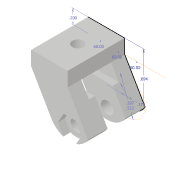
# Autodesk Inventor part: omni wheel wheel holder tilted
Saved by Autodesk Inventor 2018 (Build 220112000, 112)
## iProperties
Created: 2019-01-03
Part Number: omni wheel wheel holder tilted
Material: Generic
Document SubType Name: Modeling
Designer: ball
Density: 1 g/cm^3
Appearance: Default
Author: ball
Autodesk Inventor part; units mm, degrees
ref_plane "YZ Plane" through (0, 0, 0) normal (1, 0, 0) x (0, 1, 0)
ref_plane "XZ Plane" through (0, 0, 0) normal (0, 1, 0) x (-1, 0, 0)
ref_plane "XY Plane" through (0, 0, 0) normal (0, 0, 1) x (1, 0, 0)
sketch "Sketch1" plane through (0, 0, 0) normal (0, 0, 1) x (1, 0, 0)
  line L0 (6.5024, 17.6276) -> (-6.5024, 17.6276)
  line L1 (-6.5024, 12.5476) -> (6.5024, 12.5476) construction
  line L2 (6.5024, 12.5476) -> (13.7468, 0)
  line L3 (6.5024, 12.5476) -> (20.9911, 12.5476) construction
  line L4 (-6.5024, 12.5476) -> (0.742, 0)
  line L5 (-6.5024, 12.5476) -> (7.9863, 12.5476) construction
  line L6 (0, 12.5476) -> (7.2444, 0) construction
  line L7 (0, 12.5476) -> (14.4887, 12.5476) construction
  circle A0 centre (7.2444, 0) radius 2.1844
  circle A1 centre (7.2444, 0) radius 3.7719
  circle A2 centre (7.2444, 0) radius 6.5024 construction
  arc A3 (0.742, 0) -> (13.7468, 0) centre (7.2444, 3.7542) ccw
  line L8 (-6.5024, 17.6276) -> (-6.5024, 12.5476)
  line L9 (6.5024, 17.6276) -> (6.5024, 12.5476)
  point P0 (0, 0)
  dimension "d11" = 17.6276
  dimension "d37" = 5.08
  dimension "d38" = 60
  dimension "d39" = 60
  dimension "d40" = 60
  dimension "d41" = 4.3688
  dimension "d42" = 7.5438
  dimension "d43" = 13.0048
  constraints: 20 end point, 4 centre point, 3 equal length, 3 horizontal, 2 coincident, 2 point on circle, 1 parallel, 1 point on line, 1 vertical
  measures "d11" distance from line of L0 point (0, 0)
  measures "d37" distance between parallel lines of L1 L0
  measures "d38" angle of L2 L3
  measures "d39" angle of L4 L5
  measures "d40" angle of L6 L7
  measures "d41" diameter of A0
  measures "d42" diameter of A1
  measures "d43" diameter of A2
extrude "Extrusion1" add sketch "Sketch1" along normal blind 20.32 contours L9 L2 A3 A1 L4 L8 L0 | A3 A1 | A0 picked at (10.4509, 0.2998)
sketch "Sketch3" plane through (-6.5024, 17.6276, 0) normal (0, 1, 0) x (1, 0, 0)
  line L0 (6.6548, -14.4145) -> (6.6548, -20.32) construction
  line L1 (13.0048, 0) -> (0, 0) construction
  line L2 (6.5024, 0) -> (6.5024, -20.32) construction
  line L3 (13.0048, -20.32) -> (0, -20.32) construction
  line L4 (13.0048, 0) -> (13.0048, -20.32) construction
  line L5 (13.0048, -10.16) -> (0, -10.16) construction
  line L6 (0, 0) -> (0, -20.32) construction
  circle A0 centre (6.5024, -10.16) radius 1.9685 construction
  point P0 (6.5024, 0)
  dimension "d21" = 6.5024
  dimension "d22" = 10.16
  dimension "d23" = 3.937
  constraints: 5 midpoint, 4 end point, 1 centre point, 1 vertical
  measures "d21" distance between parallel lines of L2 L4
  measures "d22" distance between parallel lines of L5 L3
  measures "d23" diameter of A0
hole "Hole1" at (0, 17.6276, 10.16) direction (0, -1, 0) diameter 3.937 end through all
sketch "Sketch7" plane through (-6.5024, 12.5476, 0) normal (-1, 0, 0) x (0, 0, 1)
  line L0 (0, 5.08) -> (20.32, 5.08) construction
  line L1 (10.16, 5.08) -> (10.16, -16.3018) construction
  line L2 (0, -16.3018) -> (20.32, -16.3018) construction
  line L3 (0, 0) -> (20.32, 0) projected
  line L4 (10.16, 0) -> (15.494, 0)
  line L5 (10.16, 0) -> (4.826, 0)
  line L6 (4.826, 0) -> (4.826, -4.7752)
  line L7 (15.494, 0) -> (15.494, -4.7752)
  line L8 (10.16, -16.3018) -> (6.985, -16.3018)
  line L9 (10.16, -16.3018) -> (13.335, -16.3018)
  line L10 (6.985, -16.3018) -> (6.985, -4.7752)
  line L11 (6.985, -4.7752) -> (4.826, -4.7752)
  line L12 (13.335, -16.3018) -> (13.335, -4.7752)
  line L13 (13.335, -4.7752) -> (15.494, -4.7752)
  point P0 (0, -12.5476)
  dimension "d47" = 5.334
  dimension "d48" = 5.334
  dimension "d49" = 4.7752
  dimension "d50" = 4.7752
  dimension "d51" = 3.175
  dimension "d52" = 3.175
  constraints: 22 end point, 5 point on line, 3 midpoint, 3 vertical, 2 perpendicular
  measures "d47" distance of L4.start L4.end
  measures "d48" distance of L4.start L5.end
  measures "d49" distance of L5.end L6.end
  measures "d50" distance of L4.end L7.end
  measures "d51" distance of L1.end L8.end
  measures "d52" distance of L1.end L9.end
extrude "Extrusion5" cut sketch "Sketch7" against normal through all
extrude "Extrusion6" cut sketch "Sketch1" along normal blind 2.54 contours A3 A1 | A1 A3 | A0
extrude "Extrusion7" cut sketch "Sketch1" along normal through all contours A0
sketch "Sketch8" plane through (0, 0, 20.32) normal (0, 0, 1) x (1, 0, 0)
  circle A0 centre (7.2444, 0) radius 2.1844 construction
  circle A1 centre (7.2444, 0) radius 4.2545 construction
  line L0 (11.4989, 0) -> (9.0425, -4.2545)
  line L1 (5.4462, -4.2545) -> (2.9899, 0)
  line L2 (2.9899, 0) -> (5.1171, 3.6845)
  line L3 (5.1171, 3.6845) -> (9.3716, 3.6845)
  line L4 (9.3716, 3.6845) -> (11.4989, 0)
  line L5 (5.4462, -4.2545) -> (9.0425, -4.2545)
  point P0 (0, 0)
  point P1 (9.3716, -3.6845)
  point P2 (5.1171, -3.6845)
  dimension "d59" = 8.509
  constraints: 12 end point, 2 coincident, 2 point on line, 1 horizontal, 1 horizontal alignment, 13 other
extrude "Extrusion8" cut sketch "Sketch8" against normal blind 2.54
body "Solid1"
